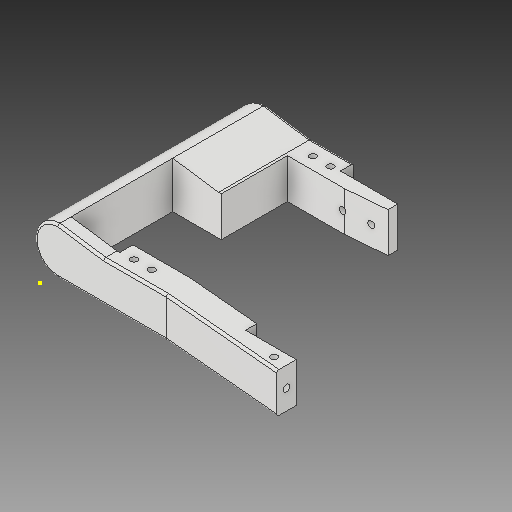
# Autodesk Inventor part: Hand - Frame
Saved by Autodesk Inventor 2017 (Build 210142000, 142)
## iProperties
Created: 2016-09-27
Part Number: Hand - Frame
Material: ABS Plastic
Document SubType Name: Modeling
Designer: cmcdona
Density: 1.06 g/cm^3
Appearance: Smooth - White
Author: cmcdona
Autodesk Inventor part; units mm, degrees
ref_plane "YZ Plane" through (0, 0, 0) normal (1, 0, 0) x (0, 1, 0)
ref_plane "XZ Plane" through (0, 0, 0) normal (0, 1, 0) x (-1, 0, 0)
sketch "Sketch1" plane through (0, 0, 0) normal (0, 0, 1) x (1, 0, 0)
  line L0 (0, 0) -> (104, 0)
  line L1 (104, 0) -> (104, 18)
  arc A0 (0, 21) -> (0, 0) centre (0, 10.5) ccw
  line L2 (0, 21) -> (20.7846, 18)
  line L3 (20.7846, 18) -> (104, 18)
  dimension "d0" = 104
  dimension "d1" = 18
  dimension "d2" = 21
  dimension "d3" = 10.5
  dimension "d4" = 21
  constraints: 8 end point, 2 perpendicular, 2 point on circle, 1 centre point, 1 horizontal
  measures "d0" distance of L0.start L0.end
  measures "d1" distance of L0.end L1.end
  measures "d2" distance of L0.start L2.start
  measures "d3" radius of A0
  measures "d4" distance of L2.start L2.end
extrude "Extrusion1" add sketch "Sketch1" against normal blind 102
sketch "Sketch2" plane through (0, 0, 0) normal (0, -1, 0) x (1, 0, 0)
  line L0 (0, 0) -> (-10.5, 0) projected
  line L1 (-10.5, 0) -> (-10.5, -8)
  line L2 (-10.5, -8) -> (49, -8)
  line L3 (49, -8) -> (140.4404, 0)
  line L4 (49, -8) -> (140.7897, -8) construction
  line L5 (140.4404, 0) -> (-10.5, 0)
  dimension "d7" = 8
  dimension "d8" = 59.5
  dimension "d9" = 5
  constraints: 10 end point, 1 collinear, 1 equal length, 1 horizontal, 1 perpendicular, 1 vertical
  measures "d7" distance of L0.end L1.end
  measures "d8" distance of L1.end L2.end
  measures "d9" angle of L4 L3
extrude "Extrusion2" cut sketch "Sketch2" against normal through all
sketch "Sketch3" plane through (0, 0, -102) normal (0, -1, 0) x (1, 0, 0)
  line L0 (22, 88) -> (22, 82)
  line L1 (0, 94) -> (0, 0) projected
  line L2 (22, 82) -> (48, 82)
  line L3 (48, 82) -> (83.863, 85.1376)
  line L4 (83.863, 85.1376) -> (91.363, 72.1472)
  line L5 (22, 88) -> (0, 88)
  line L6 (0, 88) -> (0, 42)
  line L7 (0, 42) -> (22, 42)
  line L8 (20.7846, 94) -> (20.7846, 0) projected
  line L9 (0, 42) -> (22, 42) construction
  line L10 (22, 42) -> (22, 12)
  line L11 (22, 12) -> (48, 12)
  line L12 (48, 12) -> (83.863, 8.8624)
  line L13 (83.863, 8.8624) -> (91.363, 21.8528)
  line L14 (91.363, 72.1472) -> (91.363, 21.8528)
  line L15 (104, 0) -> (0, 0) projected
  point P0 (0, 102)
  dimension "d12" = 6
  dimension "d13" = 26
  dimension "d14" = 36
  dimension "d15" = 175
  dimension "d16" = 15
  dimension "d17" = 115
  dimension "d18" = 22
  dimension "d19" = 46
  dimension "d20" = 22
  dimension "d21" = 0
  dimension "d22" = 30
  dimension "d23" = 90
  dimension "d24" = 26
  dimension "d25" = 36
  dimension "d26" = 175
  dimension "d27" = 15
  dimension "d28" = 115
  constraints: 26 end point, 4 perpendicular, 2 parallel, 2 point on line, 1 collinear, 1 horizontal
  measures "d12" distance of L0.start L0.end
  measures "d13" distance of L0.end L2.end
  measures "d14" distance of L2.end L3.end
  measures "d15" angle of L3 L2
  measures "d16" distance of L3.end L4.end
  measures "d17" angle of L3 L4
  measures "d18" distance of L0.start L5.end
  measures "d19" distance of L5.end L6.end
  measures "d20" distance of L6.end L7.end
  measures "d21" distance between parallel lines of L7 L9
  measures "d22" distance of L7.end L10.end
  measures "d23" angle of L7 L10
  measures "d24" distance of L10.end L11.end
  measures "d25" distance of L11.end L12.end
  measures "d26" angle of L11 L12
  measures "d27" distance of L12.end L13.end
  measures "d28" angle of L13 L12
extrude "Extrusion3" cut sketch "Sketch3" against normal through all contours L0 L2 L3 L4 L14 L13 L12 L11 L10 L7 L8 L5 | L8 L7 L1 L5
ref_plane "Work Plane1" through (0, 0, -96) normal (0, 0, -1) x (-1, 0, 0)
sketch "Sketch4" plane through (0, 0, -96) normal (0, 0, -1) x (-1, 0, 0)
  line L0 (-49, 18) -> (-104, 18) projected
  line L1 (-66, 0) -> (-104, 0)
  line L2 (-104, 0) -> (-104, 18)
  line L3 (-104, 18) -> (-66, 18)
  line L4 (-66, 18) -> (-66, 0)
  point P0 (0, 0)
  dimension "d32" = 38
  constraints: 8 end point, 2 parallel, 1 horizontal, 1 perpendicular
  measures "d32" distance of L0.end L3.end
extrude "Extrusion4" cut sketch "Sketch4" against normal blind 77
sketch "Sketch5" plane through (0, 0, -102) normal (0, 0, -1) x (-1, 0, 0)
  line L0 (-45, 0) -> (-45, 18)
  line L1 (-48, 0) -> (-48, 18) projected
  line L2 (-20.7846, 18) -> (-104, 18) projected
  line L3 (-45, 18) -> (-104, 18)
  line L4 (-104, 0) -> (-104, 18) projected
  line L5 (-104, 18) -> (-104, 0)
  line L6 (-104, 0) -> (-45, 0)
  point P0 (0, 0)
  constraints: 8 end point, 2 collinear, 1 parallel, 1 perpendicular
extrude "Extrusion5" cut sketch "Sketch5" against normal blind 6
ref_plane "Work Plane2" through (0, 0, -12) normal (0, 0, -1) x (-1, 0, 0)
sketch "Sketch6" plane through (0, 0, -12) normal (0, 0, -1) x (-1, 0, 0)
  line L0 (-104, 0) -> (-104, 18) projected
  line L1 (-81, 0) -> (-104, 0)
  line L2 (-104, 0) -> (-104, 18)
  line L3 (-104, 18) -> (-81, 18)
  line L4 (-81, 18) -> (-81, 0)
  point P0 (0, 0)
  dimension "d38" = 23
  constraints: 8 end point, 2 parallel, 1 horizontal, 1 perpendicular
  measures "d38" distance of L0.end L3.end
extrude "Extrusion6" cut sketch "Sketch6" along normal through all
sketch "Sketch7" plane through (104, 0, -3.1881) normal (1, 0, 0) x (0, 0, -1)
  circle A0 centre (4.412, 9) radius 1.5
  point P0 (-3.1881, 0)
  dimension "d41" = 3
  constraints: 1 centre point
  measures "d41" diameter of A0
extrude "Extrusion7" cut sketch "Sketch7" against normal blind 6
fillet "Fillet1" radius 1 10 edges at (76.5, 18, -5.5941) (76.5, 0, -5.5941) (-10.5, 10.5, -8) (24.5, 0, -8) (34.8923, 18, -8) (10.3923, 19.5, -8) (10.3923, 19.5, -102) (32.8923, 18, -102) (22.5, 0, -102) (-10.5, 10.5, -102)
sketch "Sketch8" plane through (0, 0, -96) normal (0, 0, -1) x (-1, 0, 0)
  line L0 (-45, 0) -> (-40, 0)
  line L1 (-40, 0) -> (-40, 18)
  line L2 (-40, 18) -> (-45, 18)
  line L3 (-45, 18) -> (-45, 0)
  point P0 (0, 0)
  dimension "d45" = 5
  dimension "d46" = 18
  constraints: 8 end point, 2 parallel, 1 horizontal, 1 perpendicular
  measures "d45" distance of L2.end L1.end
  measures "d46" distance of L1.end L0.end
extrude "Extrusion8" cut sketch "Sketch8" along normal through all
sketch "Sketch9" plane through (0, 0, -96) normal (0, 0, -1) x (-1, 0, 0)
  circle A0 centre (-47, 9) radius 1.5
  circle A1 centre (-59, 9) radius 1.5
  point P0 (0, 0)
  dimension "d49" = 3
  dimension "d50" = 3
  constraints: 2 centre point
  measures "d49" diameter of A0
  measures "d50" diameter of A1
extrude "Extrusion9" cut sketch "Sketch9" against normal blind 6
sketch "Sketch10" plane through (22, 18, -20) normal (0, 1, 0) x (1, 0, 0)
  circle A0 centre (76, -12) radius 1.5
  point P0 (-22, -20)
  dimension "d54" = 3
  constraints: 1 centre point
  measures "d54" diameter of A0
extrude "Extrusion10" cut sketch "Sketch10" against normal blind 5
sketch "Sketch11" plane through (22, 18, -20) normal (0, 1, 0) x (1, 0, 0)
  circle A0 centre (6, -5.5) radius 1.5
  circle A1 centre (14, -5.5) radius 1.5
  circle A2 centre (6, 75.5) radius 1.5
  circle A3 centre (14, 75.5) radius 1.5
  point P0 (-22, -20)
  dimension "d57" = 3
  dimension "d58" = 3
  dimension "d59" = 3
  dimension "d60" = 3
  constraints: 4 centre point
  measures "d57" diameter of A0
  measures "d58" diameter of A1
  measures "d59" diameter of A2
  measures "d60" diameter of A3
extrude "Extrusion11" cut sketch "Sketch11" against normal blind 6
sketch "Sketch12" plane through (22, 0, -14) normal (0, 0, -1) x (-1, 0, 0)
  line L0 (22, 0) -> (0, 0) projected
  line L1 (0, 0) -> (22, 0)
  line L2 (22, 0) -> (22, 2)
  line L3 (22, 2) -> (0, 2)
  line L4 (0, 2) -> (0, 0)
  dimension "d63" = 22
  dimension "d64" = 2
  constraints: 8 end point, 2 parallel, 1 horizontal, 1 perpendicular
  measures "d63" distance of L3.end L2.end
  measures "d64" distance of L2.end L1.end
extrude "Extrusion12" add sketch "Sketch12" along normal blind 6
sketch "Sketch14" plane through (22, 18, -14) normal (0, 0, -1) x (-1, 0, 0)
  line L0 (0.5206, -0.64) -> (21.8133, -0.64) construction
  line L1 (21.8133, -0.64) -> (21.8133, -15.538) construction
  line L2 (21.8133, -15.538) -> (0.5206, -15.538) construction
  line L3 (0.5206, -15.538) -> (0.5206, -0.64) construction
  point P0 (22, -18)
  constraints: 2 other
sketch "Sketch15" plane through (0, 2, -14) normal (0, 1, 0) x (1, 0, 0)
  line L0 (0.0966, 5.9599) -> (21.8846, 5.9599) construction
  line L1 (21.8846, 5.9599) -> (21.8846, 0.0499) construction
  line L2 (21.8846, 0.0499) -> (0.0966, 0.0499) construction
  line L3 (0.0966, 0.0499) -> (0.0966, 5.9599) construction
  point P0 (0, -14)
  constraints: 2 other
body "Solid1"
